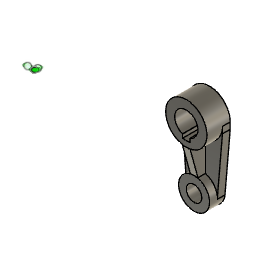
3D v1 (Autodesk Fusion 360 design; units mm, degrees)
Autodesk Fusion 360 part; units mm, degrees
sketch "Sketch1" plane through (0, 0, 0) normal (0, 1, 0) x (1, 0, 0)
  circle A0 centre (0, 0) radius 32
  circle A1 centre (0, 100) radius 24
  line L0 (32, 0) -> (32, 10)
  line L1 (32, 10) -> (23.9079, 102.1006)
  line L2 (-31.9991, 0.2374) -> (-23.9247, 101.9002)
  dimension "d1" = 64
  dimension "d2" = 48
  constraint coincident A0.centre origin
  constraint coincident A0 L0.start
  constraint tangent A0 L0
  constraint vertical L0
  constraint coincident A1 L1.end
  constraint tangent A1 L1
  constraint coincident A0 L2.start
  constraint coincident A1 L2.end
  constraint tangent A1 L2
  measures "d1" diameter of A0
  measures "d2" diameter of A1
extrude "Extrude1" add sketch "Sketch1" along normal blind 12 contours A0 A1 L0 L1 L2 makes body 1
sketch "Sketch2" plane through (0, 12, 0) normal (0, 1, 0) x (-1, 0, 0)
  line L0 (-32, -10) -> (-23.9079, -102.1006)
  arc A0 (23.9247, -101.9002) -> (-23.9079, -102.1006) centre (0, -100) ccw
  line L1 (23.9247, -101.9002) -> (31.6354, -4.8167)
  arc A1 (-32, 0) -> (31.6354, -4.8167) centre (0, 0) ccw
  line L2 (-32, 0) -> (-32, -10)
  circle A2 centre (0, 0) radius 32
  circle A3 centre (0, 0) radius 18
  constraint coincident A1.centre A2.centre
  constraint concentric A2 A3
extrude "Extrude2" add sketch "Sketch2" against normal blind 36 contours A1 A2 bodies 1
sketch "Sketch3" plane through (0, 12, 0) normal (0, 1, 0) x (-1, 0, 0)
  circle A0 centre (0, 0) radius 18
  line L0 (-32, -10) -> (-23.9079, -102.1006)
  arc A1 (23.9247, -101.9002) -> (-23.9079, -102.1006) centre (0, -100) ccw
  line L1 (23.9247, -101.9002) -> (31.6354, -4.8167)
  arc A2 (31.6354, -4.8167) -> (-32, 0) centre (0, 0) ccw
  line L2 (-32, 0) -> (-32, -10)
  circle A3 centre (0, -100) radius 24
  circle A4 centre (0, -100) radius 12
  dimension "d7" = 24
  constraint concentric A1 A3
  constraint concentric A1 A4
  measures "d7" diameter of A4
extrude "Extrude3" add sketch "Sketch3" against normal blind 24 contours A1 A3 bodies 1
sketch "Sketch4" plane through (0, 12, 0) normal (0, 1, 0) x (-1, 0, 0)
  circle A0 centre (0, -100) radius 12
  circle A1 centre (0, 0) radius 18
  line L0 (-32, -10) -> (-23.9079, -102.1006)
  arc A2 (-23.9079, -102.1006) -> (23.9247, -101.9002) centre (0, -100) ccw
  line L1 (23.9247, -101.9002) -> (31.6354, -4.8167)
  arc A3 (31.6354, -4.8167) -> (-32, 0) centre (0, 0) ccw
  line L2 (-32, 0) -> (-32, -10)
  line L3 (-5.7314, -17.0631) -> (6, -17.0631)
  line L4 (6, -17.0631) -> (6, -23)
  line L5 (6, -23) -> (-5.7314, -23)
  line L6 (-5.7314, -23) -> (-5.7314, -17.0631)
  constraint horizontal L3
  constraint vertical L4
  constraint horizontal L5
  constraint vertical L6
  constraint coincident A1 L3.start
extrude "Extrude4" cut sketch "Sketch4" against normal blind 36 contours A1 L3 L4 L5 L6 bodies 1
sketch "Sketch5" plane through (0, 0, 0) normal (1, 0, 0) x (0, 1, 0)
  line L0 (-12, -76) -> (-24, -32)
  line L1 (-24, -32) -> (0, -32)
  line L2 (0, -32) -> (0, -76)
  line L3 (0, -76) -> (-12, -76)
  constraint horizontal L1
  constraint perpendicular L1 L2
  constraint perpendicular L2 L3
extrude "Extrude5" add sketch "Sketch5" along normal blind 6 separate body makes body 2
sketch "Sketch6" plane through (0, 0, 0) normal (-1, 0, 0) x (0, -1, 0)
  line L0 (0, -32) -> (0, -76)
  line L1 (0, -76) -> (12, -76)
  line L2 (12, -76) -> (24, -32)
  line L3 (24, -32) -> (0, -32)
  line L4 (24, -32) -> (0, -32)
  line L5 (0, -76) -> (12, -76)
  constraint coincident L2.end L3.start
  constraint coincident L0.start L3.end
  constraint coincident L0.end L1.start
  constraint coincident L1.end L2.start
extrude "Extrude6" add sketch "Sketch6" along normal blind 6 bodies 2 1
sketch "Sketch7" plane through (0, 0, 0) normal (0, 0, 1) x (1, 0, 0)
  spline S0 degree 5 poles (-200, -70) (-199.5071, -70.1071) (-198.5439, -70.3047) (-197.1668, -70.5516) (-195.4683, -70.7802) (-193.5919, -70.8856) (-191.9888, -70.7912) (-190.6902, -70.4741) (-189.725, -69.9134) (-189.1054, -69.1001) (-188.8176, -68.0441) (-188.8364, -67.0173) (-188.9827, -66.1506) (-189.138, -65.5306) (-189.2301, -65.21) knots 0 0 0 0 0 0 0.1 0.2 0.3 0.4 0.5 0.6 0.7 0.8 0.9 1 1 1 1 1 1
  point P0 (-190, -70)
